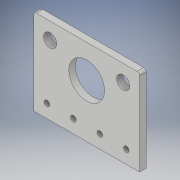
# Autodesk Inventor part: Stepper_to_rail
Saved by Autodesk Inventor 2019 (Build 230136000, 136)
## iProperties
Created: 2021-06-18
Part Number: Stepper_to_rail
Material: Generic
Document SubType Name: Modeling
Designer: 91742
Density: 1 g/cm^3
Appearance: Default
Author: 91742
Autodesk Inventor part; units mm, degrees
ref_plane "YZ Plane" through (0, 0, 0) normal (1, 0, 0) x (0, 1, 0)
ref_plane "XZ Plane" through (0, 0, 0) normal (0, 1, 0) x (-1, 0, 0)
ref_plane "XY Plane" through (0, 0, 0) normal (0, 0, 1) x (1, 0, 0)
sketch "Sketch1" plane through (0, 0, 0) normal (0, 0, 1) x (1, 0, 0)
  line L0 (38, 55) -> (0, 55)
  line L1 (-38, 55) -> (0, 55)
  arc A0 (-38, 55) -> (-40, 53) centre (-38, 53) ccw
  arc A1 (40, 53) -> (38, 55) centre (38, 53) ccw
  circle A2 centre (0, 30) radius 13.5
  circle A3 centre (27.6, 42.5) radius 5
  circle A4 centre (-27.6, 42.5) radius 5
  line L2 (-40, 2) -> (-40, 2)
  line L3 (40, 2) -> (40, 2)
  line L4 (-40, 53) -> (-40, 0)
  line L5 (40, 0) -> (40, 53)
  line L6 (-40, 0) -> (-40, -10)
  line L7 (-40, -10) -> (40, -10)
  line L8 (40, -10) -> (40, 0)
  circle A5 centre (30, 0) radius 2.1
  circle A6 centre (-30, 0) radius 2.1
  circle A7 centre (-10, 0) radius 2.1
  circle A8 centre (10, 0) radius 2.1
  point P0 (40, 55)
  dimension "d7" = 2
  dimension "d8" = 27
  dimension "d9" = 10
  dimension "d15" = 10
  dimension "d17" = 4.2
  dimension "d18" = 4.2
  dimension "d21" = 4.2
  dimension "d22" = 4.2
  dimension "d25" = 52.5
  dimension "d26" = 40
  constraints: 18 end point, 9 centre point, 5 vertical, 4 point on circle, 2 horizontal, 2 point on line, 2 tangent, 1 equal radius, 1 perpendicular
  measures "d7" radius of A0
  measures "d8" diameter of A2
  measures "d9" diameter of A3
  measures "d15" distance of L4.end L6.end
  measures "d17" diameter of A5
  measures "d18" diameter of A6
  measures "d21" diameter of A7
  measures "d22" diameter of A8
  measures "d25" distance from line of L7 A4.centre
  measures "d26" distance from line of L7 A2.centre
extrude "Extrusion3" add sketch "Sketch1" along normal blind 5
body "Solid3"
